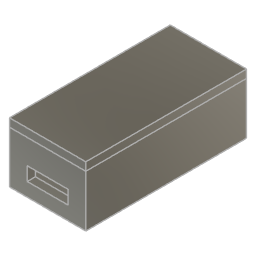
light-check-case (Autodesk Fusion 360 design; units mm, degrees)
Autodesk Fusion 360 part; units mm, degrees
sketch "Skizze1" plane through (0, 0, 0) normal (0, 0, 1) x (1, 0, 0) in component "light-on-checker"
  line L0 (0, 0) -> (-22, 0)
  line L1 (-22, 0) -> (-22, -53)
  line L2 (-22, -53) -> (0, -53)
  line L3 (0, -53) -> (0, 0)
  line L4 (3, -56) -> (3, 3)
  line L5 (3, 3) -> (-25, 3)
  line L6 (-25, 3) -> (-25, -56)
  line L7 (-25, -56) -> (3, -56)
  dimension "d11" = 22
  dimension "d12" = 53
  dimension "d13" = 3
  constraint horizontal L0
  constraint vertical L1
  constraint horizontal L2
  constraint vertical L3
  constraint coincident L0.start L3.end
  measures "d11" distance of L0.start L0.end
  measures "d12" distance of L0.start L2.end
extrude "Extrusion1" add sketch "Skizze1" along normal blind 3 contours L0 L1 L2 L3 makes body 1 in component "light-on-checker"
extrude "Extrusion2" add sketch "Skizze1" along normal blind 19 bodies 1 in component "light-on-checker"
extrude "Extrusion3" add sketch "Skizze1" along normal blind 3 from surface at 19 separate body contours L0 L1 L2 L3 | L4 L5 L6 L7 makes body 2 in component "light-on-checker"
sketch "Skizze2" plane through (0, 0, 3) normal (0, 0, 1) x (-1, 0, 0) in component "light-on-checker"
  line L0 (0, 53) -> (0, 0)
  line L1 (0, 0) -> (22, 0)
  line L2 (22, 0) -> (22, 53)
  line L3 (22, 53) -> (0, 53)
  line L4 (0, 0) -> (22, 53) construction
  line L5 (21.595, 4.91) -> (0.405, 4.91) construction
  line L6 (0.405, 4.91) -> (0.405, 48.09) construction
  line L7 (0.405, 48.09) -> (21.595, 48.09) construction
  line L8 (21.595, 48.09) -> (21.595, 4.91) construction
  line L9 (21.595, 4.91) -> (0.405, 48.09) construction
  line L10 (0.405, 4.91) -> (21.595, 48.09) construction
  line L11 (19.125, 48.09) -> (19.125, 4.91) construction
  line L12 (2.8749, 48.09) -> (2.8749, 4.8867) construction
  line L13 (19.125, 11.29) -> (2.8749, 11.29) construction
  line L14 (2.8749, 41.71) -> (19.125, 41.71) construction
  circle A0 centre (19.125, 41.71) radius 1
  circle A1 centre (2.8749, 11.29) radius 1
  point P0 (11, 26.5)
  dimension "d21" = 21.19
  dimension "d22" = 43.18
  dimension "d23" = 2.47
  dimension "d24" = 2.47
  dimension "d25" = 6.38
  dimension "d26" = 6.38
  dimension "d27" = 2
  dimension "d28" = 2
  constraint coincident L0.end L1.start
  constraint coincident L2.end L3.start
  constraint horizontal L5
  constraint perpendicular L5 L6
  constraint parallel L5 L7
  constraint parallel L6 L8
  constraint coincident L9 P0
  constraint coincident L10 P0
  constraint midpoint L4 P0
  constraint coincident L7 L11.start
  constraint coincident L5 L11.end
  constraint perpendicular L5 L11
  constraint coincident L7 L12.start
  constraint perpendicular L7 L12
  constraint coincident L11 L13.start
  constraint coincident L12 L13.end
  constraint perpendicular L12 L13
  constraint coincident L12 L14.start
  constraint coincident L11 L14.end
  constraint perpendicular L11 L14
  constraint coincident L14.end A0.centre
  constraint coincident L13.end A1.centre
  measures "d21" distance of L6.end L7.end
  measures "d22" distance of L5.end L6.end
  measures "d23" distance of L5.start L11.end
  measures "d24" distance of L5.end L12.end
  measures "d25" distance of L11.start L14.end
  measures "d26" distance of L11.end L13.start
  measures "d27" diameter of A0
  measures "d28" diameter of A1
extrude "Extrusion4" cut sketch "Skizze2" against normal blind 7 contours A0 | A1 bodies 1 in component "light-on-checker"
sketch "Skizze3" plane through (0, 3, 0) normal (0, 1, 0) x (-1, 0, 0) in component "light-on-checker"
  line L0 (-3, 0) -> (25, 0)
  line L1 (25, 0) -> (25, 19)
  line L2 (25, 19) -> (-3, 19)
  line L3 (-3, 19) -> (-3, 0)
  circle A0 centre (17, 8) radius 2.5
  dimension "d31" = 5
  dimension "d32" = 8
  dimension "d33" = 8
  measures "d31" diameter of A0
  measures "d32" distance of L1 A0.centre
  measures "d33" distance of L0 A0.centre
extrude "Extrusion5" cut sketch "Skizze3" against normal blind 8 contours A0 bodies 1 in component "light-on-checker"
sketch "Skizze4" plane through (0, -56, 0) normal (0, -1, 0) x (1, 0, 0) in component "light-on-checker"
  line L0 (-25, 0) -> (3, 0)
  line L1 (3, 0) -> (3, 19)
  line L2 (3, 19) -> (-25, 19)
  line L3 (-25, 19) -> (-25, 0)
  line L4 (-18.5, 10) -> (-3.5, 10)
  line L5 (-3.5, 10) -> (-3.5, 5)
  line L6 (-3.5, 5) -> (-18.5, 5)
  line L7 (-18.5, 5) -> (-18.5, 10)
  line L8 (-25, 5) -> (3, 5) construction
  dimension "d36" = 15
  dimension "d37" = 5
  dimension "d38" = 5
  constraint horizontal L4
  constraint vertical L5
  constraint horizontal L6
  constraint vertical L7
  constraint coincident L3 L8.start
  constraint coincident L1 L8.end
  constraint perpendicular L1 L8
  constraint midpoint L6 L8
  measures "d36" distance of L4.start L4.end
  measures "d37" distance of L4.start L6.end
  measures "d38" distance of L0.end L8.end
extrude "Extrusion6" cut sketch "Skizze4" against normal blind 9 contours L4 L5 L6 L7 bodies 1 in component "light-on-checker"
component "light-on-checker" placed x (1, 0, 0) y (0, 1, 0) z (0, 0, 1) at (0, 0, 0)
equation "d16 = 3.00 mm + 16 mm"
equation "d114 = 2 mm + 25.4 mm"
